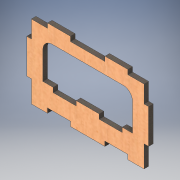
# Autodesk Inventor part: stiffenerFront
Saved by Autodesk Inventor 2019 (Build 230136000, 136)
## iProperties
Created: 2020-12-06
Part Number: stiffenerFront
Material: Дерево (береза)
Document SubType Name: Modeling
Designer: Professional
Density: 0.55 g/cm^3
Appearance: Береза — натуральный — полированный
Author: Professional
Autodesk Inventor part; units mm, degrees
ref_plane "YZ Plane" through (0, 0, 0) normal (1, 0, 0) x (0, 1, 0)
ref_plane "XZ Plane" through (0, 0, 0) normal (0, 1, 0) x (-1, 0, 0)
ref_plane "XY Plane" through (0, 0, 0) normal (0, 0, 1) x (1, 0, 0)
sketch "Эскиз1" plane through (0, 0, 0) normal (0, 0, 1) x (1, 0, 0)
  line L0 (0, 0) -> (0, 64) construction
  line L1 (0, 64) -> (-15, 64)
  line L2 (-15, 64) -> (-15, 68)
  line L3 (-15, 68) -> (-35, 68)
  line L4 (-35, 68) -> (-35, 64)
  line L5 (-35, 64) -> (-49, 64)
  line L6 (-49, 64) -> (-49, 49)
  line L7 (-49, 49) -> (-53, 49)
  line L8 (-53, 49) -> (-53, 19)
  line L9 (-53, 19) -> (-49, 19)
  line L10 (-49, 19) -> (-49, 0)
  line L11 (-39, 22) -> (-39, 54)
  line L12 (0, 0) -> (-15, 0)
  line L13 (-15, 0) -> (-15, 4)
  line L14 (-15, 4) -> (-35, 4)
  line L15 (-35, 4) -> (-35, 0)
  line L16 (-35, 0) -> (-49, 0)
  line L17 (-39, 22) -> (-30, 22)
  line L18 (-30, 22) -> (-30, 18)
  line L19 (-30, 18) -> (-10, 18)
  line L20 (-10, 18) -> (-10, 22)
  line L21 (-10, 22) -> (0, 22)
  line L22 (-39, 54) -> (0, 54)
  line L23 (0, 64) -> (15, 64)
  line L24 (15, 64) -> (15, 68)
  line L25 (15, 68) -> (35, 68)
  line L26 (35, 68) -> (35, 64)
  line L27 (35, 64) -> (49, 64)
  line L28 (49, 64) -> (49, 49)
  line L29 (49, 49) -> (53, 49)
  line L30 (53, 49) -> (53, 19)
  line L31 (53, 19) -> (49, 19)
  line L32 (49, 19) -> (49, 0)
  line L33 (39, 22) -> (39, 54)
  line L34 (0, 0) -> (15, 0)
  line L35 (15, 0) -> (15, 4)
  line L36 (15, 4) -> (35, 4)
  line L37 (35, 4) -> (35, 0)
  line L38 (35, 0) -> (49, 0)
  line L39 (39, 22) -> (30, 22)
  line L40 (30, 22) -> (30, 18)
  line L41 (30, 18) -> (10, 18)
  line L42 (10, 18) -> (10, 22)
  line L43 (10, 22) -> (0, 22)
  line L44 (39, 54) -> (0, 54)
  point P0 (0, 32)
  point P1 (53, 32)
  dimension "d0" = 30
  dimension "d8" = 10
  dimension "d12" = 4
  dimension "d13" = 18
  dimension "d14" = 20
  dimension "d15" = 20
  dimension "d16" = 68
  dimension "d17" = 30
  dimension "d18" = 20
  dimension "d19" = 10
  dimension "d20" = 78
  dimension "d21" = 30
  dimension "d22" = 20
  dimension "d23" = 19
  constraints: 90 end point, 20 symmetric about line, 18 point on line, 15 perpendicular, 3 equal length, 2 horizontal, 1 midpoint, 1 vertical
  measures "d0" distance of L7.end L8.end
  measures "d8" distance between parallel lines of L10 L11
  measures "d12" distance of L8.end L9.end
  measures "d13" distance from line of L11.start L14
  measures "d14" distance between parallel lines of L20 L18
  measures "d15" distance between parallel lines of L13 L15
  measures "d16" distance between parallel lines of L3 L16
  measures "d17" diameter of L13 L0
  measures "d18" diameter of L20 L0
  measures "d19" distance between parallel lines of L1 L22
  measures "d20" diameter of L11 L0
  measures "d21" diameter of L2 L0
  measures "d22" distance between parallel lines of L2 L4
  measures "d23" distance between parallel lines of L16 L9
extrude "Выдавливание1" add sketch "Эскиз1" along normal blind 4
fillet "Сопряжение1" radius 8 2 edges at (-39, 54, 2) (39, 54, 2)
